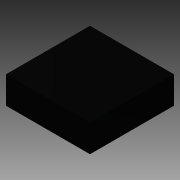
# Autodesk Inventor part: LTC3105EDDPBF
Saved by Autodesk Inventor 2015 SP1 (Build 190203100, 203)
## iProperties
Created: 2015-10-19
Part Number: LTC3105EDDPBF
Material: Generic
Document SubType Name: Modeling
Designer: Kartikye
Density: 1 g/cm^3
Appearance: DFN300X300X80-11N, LTC3105EDDPBF
Author: Kartikye
Autodesk Inventor part; units mm, degrees
ref_plane "YZ Plane" through (0, 0, 0) normal (1, 0, 0) x (0, 1, 0)
ref_plane "XZ Plane" through (0, 0, 0) normal (0, 1, 0) x (-1, 0, 0)
ref_plane "XY Plane" through (0, 0, 0) normal (0, 0, 1) x (1, 0, 0)
sketch "DFN300X300X80-11N, LTC3105EDDPBF_102" plane through (0, 0, 0) normal (0, 0, 1) x (1, 0, 0)
  line L0 (-1.4986, 1.4986) -> (1.5748, 1.4986)
  line L1 (1.5748, 1.4986) -> (1.5748, -1.5748)
  line L2 (1.5748, -1.5748) -> (-1.4986, -1.5748)
  line L3 (-1.4986, -1.5748) -> (-1.4986, 1.4986)
  constraints: 8 end point
extrude "Extrusion1" add sketch "DFN300X300X80-11N, LTC3105EDDPBF_102" along normal blind 1
body "Solid1"
